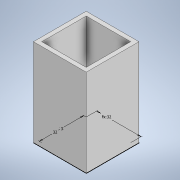
# Autodesk Inventor part: single
Saved by Autodesk Inventor 2022 (Build 260153000, 153)
## iProperties
Created: 2021-10-08
Part Number: single
Material: Generic
Document SubType Name: Modeling
Designer: dangl
Density: 1 g/cm^3
Appearance: Default
Author: dangl
Autodesk Inventor part; units mm, degrees
ref_plane "YZ Plane" through (0, 0, 0) normal (1, 0, 0) x (0, 1, 0)
ref_plane "XZ Plane" through (0, 0, 0) normal (0, 1, 0) x (-1, 0, 0)
ref_plane "XY Plane" through (0, 0, 0) normal (0, 0, 1) x (1, 0, 0)
sketch "Sketch1" plane through (0, 0, 0) normal (0, 1, 0) x (-1, 0, 0)
  line L0 (0, 0) -> (32, 0)
  line L1 (32, 0) -> (32, -32)
  line L2 (32, -32) -> (0, -32)
  line L3 (0, -32) -> (0, 0)
  line L4 (0, -32) -> (0, 0)
  line L5 (35, -35) -> (35, 3)
  line L6 (35, 3) -> (-3, 3)
  line L7 (-3, 3) -> (-3, -35)
  line L8 (-3, -35) -> (35, -35)
  point P0 (0, -33)
  point P1 (0, -37)
  point P2 (0, 4)
  dimension "d0" = 32
  dimension "d1" = 32
  dimension "d5" = 3
  constraints: 18 end point, 4 parallel, 2 perpendicular, 1 horizontal, 1 point on line, 3 other
  measures "d0" distance of L0.end L1.end
  measures "d1" distance of L2.end L1.end
  measures "d5" distance between parallel lines of L1 L5
extrude "Extrusion1" add sketch "Sketch1" along normal blind 3 contours L0 L1 L2 L3 | L8 L7 L6 L5
extrude "Extrusion4" add sketch "Sketch1" along normal blind 63
equation "\"d1\" = d0"
body "Solid1"
